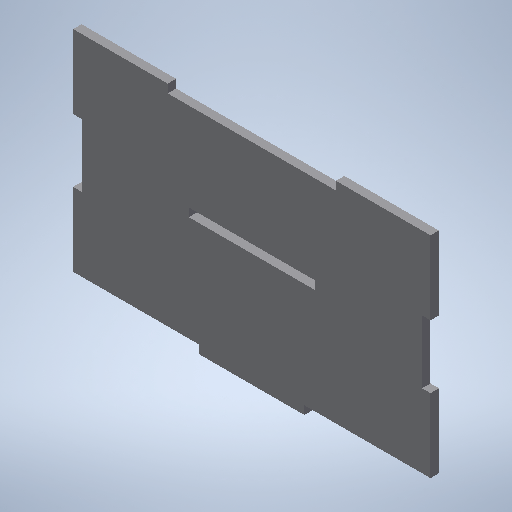
# Autodesk Inventor part: Tapa Tracera
Saved by Autodesk Inventor 2025 (Build 290162000, 162)
## iProperties
Created: 2024-10-18
Part Number: Tapa Tracera
Material: Generic
Document SubType Name: Modeling
Designer: feder
Density: 1 g/cm^3
Appearance: Default
Author: feder
Autodesk Inventor part; units mm, degrees
ref_plane "YZ Plane" through (0, 0, 0) normal (1, 0, 0) x (0, 1, 0)
ref_plane "XZ Plane" through (0, 0, 0) normal (0, 1, 0) x (-1, 0, 0)
ref_plane "XY Plane" through (0, 0, 0) normal (0, 0, 1) x (1, 0, 0)
sketch "Sketch1" plane through (0, 0, 0) normal (0, 0, 1) x (1, 0, 0)
  line L0 (-85, 0) -> (85, 0)
  line L1 (85, 0) -> (85, 100)
  line L2 (85, 100) -> (-85, 100)
  line L3 (-85, 100) -> (-85, 0)
  point P0 (0, 0)
  point P1 (0, 0)
  dimension "d0" = 170
  dimension "d1" = 100
  constraints: 8 end point, 2 coincident, 2 parallel, 1 horizontal, 1 midpoint, 1 perpendicular
  measures "d0" distance of L1.end L2.end
  measures "d1" distance of L0.end L1.end
extrude "Extrusion1" add sketch "Sketch1" along normal blind 4
sketch "Sketch2" plane through (-85, 0, 0) normal (0, -1, 0) x (1, 0, 0)
  line L0 (170, 4) -> (0, 4) projected
  line L1 (170, 0) -> (0, 0) projected
  line L2 (60, 4) -> (110, 4)
  line L3 (110, 4) -> (110, 0)
  line L4 (110, 0) -> (60, 0)
  line L5 (60, 0) -> (60, 4)
  point P0 (85, 0)
  point P1 (85, 0)
  dimension "d4" = 25
  dimension "d5" = 50
  constraints: 8 end point, 2 parallel, 2 point on line, 1 horizontal, 1 midpoint, 1 perpendicular
  measures "d4" distance from line of L3 point (85, 0)
  measures "d5" distance between parallel lines of L5 L3
extrude "Extrusion2" add sketch "Sketch2" along normal blind 4
sketch "Sketch4" plane through (0, 0, 4) normal (0, 0, 1) x (1, 0, 0)
  line L0 (85, 0) -> (85, 100) projected
  line L1 (85, 35) -> (81, 35)
  line L2 (81, 35) -> (81, 65)
  line L3 (81, 65) -> (85, 65)
  line L4 (85, 65) -> (85, 35)
  line L5 (85, 100) -> (-85, 100) projected
  line L6 (25, 0) -> (85, 0) projected
  point P0 (0, 0)
  dimension "d12" = 4
  dimension "d13" = 35
  dimension "d14" = 35
  constraints: 8 end point, 2 parallel, 1 horizontal, 1 perpendicular, 1 point on line
  measures "d12" distance of L2.end L3.end
  measures "d13" distance between parallel lines of L3 L5
  measures "d14" distance between parallel lines of L6 L1
extrude "Extrusion4" cut sketch "Sketch4" against normal blind 10
mirror "Mirror2" about plane through (0, 0, 0) normal (1, 0, 0) of "Extrusion4"
sketch "Sketch5" plane through (-85, 100, 0) normal (0, 1, 0) x (1, 0, 0)
  line L0 (170, -4) -> (0, -4) projected
  line L1 (45, 0) -> (125, 0)
  line L2 (125, 0) -> (125, -4)
  line L3 (125, -4) -> (45, -4)
  line L4 (45, -4) -> (45, 0)
  line L5 (170, 0) -> (0, 0) projected
  point P0 (85, 0)
  point P1 (85, 0)
  point P2 (45, -4)
  dimension "d17" = 80
  dimension "d18" = 40
  constraints: 8 end point, 2 parallel, 1 horizontal, 1 midpoint, 1 perpendicular, 1 point on line
  measures "d17" distance of L1.start L1.end
  measures "d18" distance from line of L2 point (85, 0)
extrude "Extrusion5" cut sketch "Sketch5" against normal blind 4
sketch "Sketch6" plane through (0, 0, 4) normal (0, 0, 1) x (1, 0, 0)
  line L0 (-30, 54) -> (30, 54)
  line L1 (30, 54) -> (30, 50)
  line L2 (30, 50) -> (-30, 50)
  line L3 (-30, 50) -> (-30, 54)
  point P0 (0, 0)
  point P1 (0, 54)
  dimension "d21" = 60
  dimension "d22" = 4
  dimension "d23" = 50
  constraints: 8 end point, 2 parallel, 1 horizontal, 1 midpoint, 1 perpendicular, 1 vertical alignment
  measures "d21" distance of L0.start L0.end
  measures "d22" distance of L0.end L1.end
  measures "d23" distance from line of point (0, 0) L2
extrude "Extrusion6" cut sketch "Sketch6" against normal blind 10
body "Solid1"
